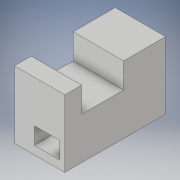
# Autodesk Inventor part: Model Creation 2
Saved by Autodesk Inventor 2019 (Build 230136000, 136)
## iProperties
Created: 2019-09-09
Part Number: Model Creation 2
Material: Generic
Document SubType Name: Modeling
Designer: IED8
Density: 1 g/cm^3
Appearance: Default
Author: IED8
Autodesk Inventor part; units mm, degrees
ref_plane "YZ Plane" through (0, 0, 0) normal (1, 0, 0) x (0, 1, 0)
ref_plane "XZ Plane" through (0, 0, 0) normal (0, 1, 0) x (-1, 0, 0)
ref_plane "XY Plane" through (0, 0, 0) normal (0, 0, 1) x (1, 0, 0)
sketch "Sketch1" plane through (0, 0, 0) normal (1, 0, 0) x (0, 1, 0)
  line L0 (0, 0) -> (0, -60)
  line L1 (0, -60) -> (40, -60)
  line L2 (40, -60) -> (40, -35)
  line L3 (40, -35) -> (25, -35)
  line L4 (25, -35) -> (25, -10)
  line L5 (25, -10) -> (40, -10)
  line L6 (40, -10) -> (40, 0)
  line L7 (40, 0) -> (0, 0)
  dimension "d0" = 60
  dimension "d1" = 40
  dimension "d2" = 25
  dimension "d3" = 15
  dimension "d4" = 25
  constraints: 16 end point, 5 perpendicular, 2 point on line, 1 parallel, 1 vertical
  measures "d0" distance of L0.start L0.end
  measures "d1" distance of L0.end L1.end
  measures "d2" distance of L1.end L2.end
  measures "d3" distance of L2.end L3.end
  measures "d4" distance of L3.end L4.end
extrude "Extrusion1" add sketch "Sketch1" along normal blind 30
sketch "Sketch2" plane through (0, 0, -60) normal (0, 0, -1) x (-1, 0, 0)
  line L0 (-30, 40) -> (-30, 0) projected
  line L1 (-30, 0) -> (-30, 5)
  line L2 (-27, 5) -> (-27, 15)
  line L3 (-27, 15) -> (-12, 15)
  line L4 (-12, 15) -> (-12, 5)
  line L5 (-12, 5) -> (-27, 5)
  point P0 (0, 0)
  dimension "d7" = 5
  dimension "d8" = 3
  dimension "d9" = 10
  dimension "d10" = 15
  constraints: 10 end point, 3 perpendicular, 1 point on line
  measures "d7" distance of L0.end L1.end
  measures "d8" distance of L1.end L2.start
  measures "d9" distance of L2.start L2.end
  measures "d10" distance of L2.end L3.end
extrude "Extrusion2" cut sketch "Sketch2" against normal blind 60
body "Solid1"
